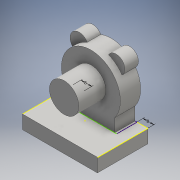
# Autodesk Inventor part: 240626_part2
Saved by Autodesk Inventor 2016 (Build 200138000, 138)
## iProperties
Created: 2024-06-26
Part Number: 240626_part2
Material: 일반
Document SubType Name: Modeling
Designer: pc
Density: 1 g/cm^3
Appearance: 기본값
Author: pc
Autodesk Inventor part; units mm, degrees
ref_plane "YZ Plane" through (0, 0, 0) normal (1, 0, 0) x (0, 1, 0)
ref_plane "XZ Plane" through (0, 0, 0) normal (0, 1, 0) x (-1, 0, 0)
ref_plane "XY Plane" through (0, 0, 0) normal (0, 0, 1) x (1, 0, 0)
sketch "스케치1" plane through (0, 0, 0) normal (0, 0, 1) x (1, 0, 0)
  line L0 (27.7299, -18.5773) -> (-27.7299, -18.5773)
  line L1 (-27.7299, -18.5773) -> (-27.7299, 18.5773)
  line L2 (-27.7299, 18.5773) -> (27.7299, 18.5773)
  line L3 (27.7299, 18.5773) -> (27.7299, -18.5773)
  line L4 (27.7299, -18.5773) -> (-27.7299, 18.5773) construction
  line L5 (-27.7299, -18.5773) -> (27.7299, 18.5773) construction
  point P0 (0, 0)
  constraints: 12 end point, 2 midpoint, 2 parallel, 1 horizontal, 1 perpendicular
extrude "돌출1" add sketch "스케치1" along normal blind 10
sketch "스케치2" plane through (0, 0, 10) normal (0, 0, 1) x (1, 0, 0)
  line L0 (27.7299, 18.5773) -> (-27.7299, 18.5773) projected
  line L1 (-19.7299, 18.5773) -> (19.7299, 18.5773)
  line L2 (19.7299, 18.5773) -> (19.7299, 3.5485)
  line L3 (19.7299, 3.5485) -> (-19.7299, 3.5485)
  line L4 (-19.7299, 3.5485) -> (-19.7299, 18.5773)
  line L5 (27.7299, -18.5773) -> (27.7299, 18.5773) projected
  line L6 (-27.7299, 18.5773) -> (-27.7299, -18.5773) projected
  point P0 (0, 0)
  dimension "d2" = 8
  dimension "d3" = 8
  constraints: 8 end point, 2 parallel, 1 horizontal, 1 perpendicular, 1 point on line
  measures "d2" distance between parallel lines of L5 L2
  measures "d3" distance between parallel lines of L6 L4
sketch "스케치3" plane through (-27.7299, 18.5773, 0) normal (0, 1, 0) x (1, 0, 0)
  line L0 (0, -10) -> (55.4598, -10) projected
  line L1 (46.066, -10) -> (10.9091, -10)
  line L2 (10.9091, -10) -> (10.9091, -19.7265)
  line L3 (10.9091, -19.7265) -> (46.066, -19.7265)
  line L4 (46.066, -19.7265) -> (46.066, -10)
  circle A0 centre (28.4876, -32.3685) radius 21.7725
  point P0 (27.7299, 0)
  constraints: 8 end point, 2 parallel, 1 centre point, 1 horizontal, 1 perpendicular, 1 point on line
extrude "돌출2" add sketch "스케치3" against normal blind 15
sketch "스케치4" plane through (-27.7299, 3.5773, 0) normal (0, -1, 0) x (1, 0, 0)
  circle A0 centre (28.6894, 33.7874) radius 10.835
  arc A1 (46.066, 19.5217) -> (10.9091, 19.5217) centre (28.4876, 32.3685) ccw projected
  arc A2 (46.2263, 44.9931) -> (36.5571, 52.5904) centre (41.9392, 49.4885) ccw
  arc A3 (21.0294, 52.8238) -> (10.3775, 44.4543) centre (15.036, 49.4885) ccw
  point P0 (27.7299, 0)
  constraints: 10 point on circle, 3 centre point
extrude "돌출3" add sketch "스케치4" along normal blind 20 contours A0
sketch "스케치5" plane through (-27.7299, 18.5773, 0) normal (0, 1, 0) x (1, 0, 0)
  arc A0 (10.9091, -19.5217) -> (46.066, -19.5217) centre (28.4876, -32.3685) ccw projected
  arc A1 (10.2823, -44.3105) -> (20.7748, -52.7291) centre (14.8621, -49.3505) ccw
  arc A2 (36.5162, -52.6067) -> (46.5049, -44.5922) centre (42.1131, -49.3505) ccw
  point P0 (27.7299, 0)
  constraints: 10 point on circle, 2 centre point
extrude "돌출4" add sketch "스케치5" against normal blind 10
